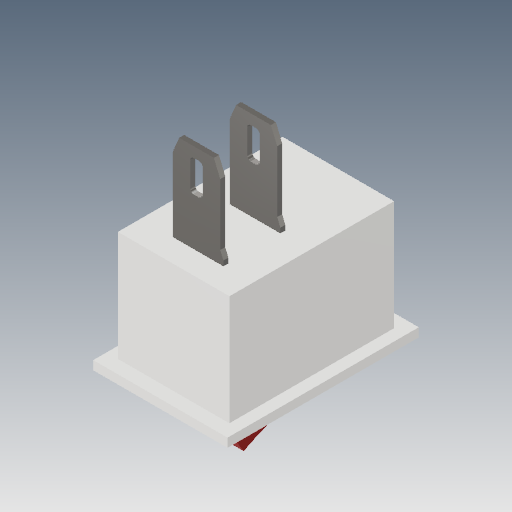
# Autodesk Inventor part: switch_6A
Saved by Autodesk Inventor 2018 (Build 220112000, 112)
## iProperties
Created: 2018-03-28
Part Number: switch_6A
Material: 一般
Document SubType Name: Modeling
Designer: y6tada
Density: 1 g/cm^3
Appearance: 既定
Sending System: SolidWorks 2017
Last Author: y6tada
Last Saved: 2018-06-10
Author: y6tada
Autodesk Inventor part; units mm, degrees
ref_plane "YZ Plane" through (0, 0, 0) normal (1, 0, 0) x (0, 1, 0)
ref_plane "XZ Plane" through (0, 0, 0) normal (0, 1, 0) x (-1, 0, 0)
sketch "スケッチ1" plane through (0, 0, 0) normal (0, 1, 0) x (-1, 0, 0)
  line L0 (4.4, -6.5) -> (-4.4, -6.5)
  line L1 (-4.4, -6.5) -> (-4.4, 6.5)
  line L2 (-4.4, 6.5) -> (4.4, 6.5)
  line L3 (4.4, 6.5) -> (4.4, -6.5)
  line L4 (-4.4, 0) -> (0, 0) construction
  line L5 (0, 0) -> (0, -6.5) construction
  dimension "d0" = 13
  dimension "d1" = 8.8
  constraints: 12 end point, 2 horizontal, 2 midpoint, 2 parallel, 1 perpendicular, 1 vertical
  measures "d0" distance between parallel lines of L2 L0
  measures "d1" distance between parallel lines of L3 L1
extrude "押し出し1" add sketch "スケッチ1" along normal blind 8.7
sketch "スケッチ2" plane through (0, 0, 0) normal (0, -1, 0) x (1, 0, 0)
  line L0 (5.3, 7.55) -> (-5.3, 7.55)
  line L1 (-5.3, 7.55) -> (-5.3, -7.55)
  line L2 (-5.3, -7.55) -> (5.3, -7.55)
  line L3 (5.3, -7.55) -> (5.3, 7.55)
  line L4 (5.3, 0) -> (0, 0) construction
  line L5 (0, 0) -> (0, -7.55) construction
  dimension "d4" = 15.1
  dimension "d5" = 10.6
  constraints: 12 end point, 2 horizontal, 2 midpoint, 2 parallel, 1 perpendicular, 1 vertical
  measures "d4" distance of L0.end L1.end
  measures "d5" distance of L1.end L2.end
extrude "押し出し2" add sketch "スケッチ2" along normal blind 1.5
sketch "スケッチ3" plane through (0, 0, 0) normal (0, 0, 1) x (1, 0, 0)
  line L0 (5.3, -1.5) -> (-5.3, -1.5) construction
  line L1 (-5.3, -1.5) -> (-5.3, -0.7)
  line L2 (-5.3, 0) -> (-5.3, -1.5) construction
  line L3 (-5.3, -0.7) -> (-3.6, -1.5)
  line L4 (-3.6, -1.5) -> (-5.3, -1.5)
  point P0 (0, 0)
  dimension "d8" = 1.7
  dimension "d9" = 0.8
  constraints: 6 end point, 1 perpendicular, 1 point on line
  measures "d8" distance from line of L1 L3.end
  measures "d9" distance of L0.end L1.end
sketch "スケッチ4" plane through (0, -1.5, 0) normal (0, -1, 0) x (1, 0, 0)
  line L0 (5.3, 7.55) -> (-5.3, 7.55) construction
  line L1 (-5.3, 7.55) -> (-5.3, -7.55) construction
  line L2 (-5.3, -7.55) -> (5.3, -7.55) construction
  line L3 (5.3, -7.55) -> (5.3, 7.55) construction
  line L4 (-3.6, 5.85) -> (3.6, 5.85)
  line L5 (3.6, 5.85) -> (3.6, -5.85)
  line L6 (3.6, -5.85) -> (-3.6, -5.85)
  line L7 (-3.6, -5.85) -> (-3.6, 5.85)
  point P0 (0, 0)
  dimension "d10" = 1.7
  constraints: 8 end point, 3 other
  measures "d10" distance between parallel lines of L0 L4
sweep "スイープ1" cut profiles "スケッチ3" path "スケッチ4"
sketch "スケッチ5" plane through (0, 0, 0) normal (1, 0, 0) x (0, 1, 0)
  line L0 (-1.5, 5.85) -> (-1.5, -5.85) construction
  arc A0 (-1.5, -5) -> (-3.75, 4.0973) centre (-21.0161, -5) ccw
  line L1 (-1.5, 5) -> (-1.5, -5)
  line L2 (-21.0161, -5) -> (-1.5, -5) construction
  arc A1 (-1.5, 5) -> (-3.75, 4.0973) centre (-0.8, 0) ccw
  line L3 (-0.8, 0) -> (0, 0) construction
  dimension "d16" = 2.25
  dimension "d17" = 0.8
  dimension "d18" = 10
  constraints: 6 end point, 4 point on circle, 2 centre point, 2 horizontal, 2 point on line, 1 collinear, 1 symmetric about line
  measures "d16" distance from line of L0 A0.end
  measures "d17" distance of L3.start L3.end
  measures "d18" distance of L1.end L1.start
extrude "押し出し3" add sketch "スケッチ5" along normal mid plane 6.25
sketch "スケッチ6" plane through (0, 0, 0) normal (0, 0, 1) x (1, 0, 0)
  line L0 (4.4, 8.7) -> (-4.4, 8.7) construction
  line L1 (0, 8.7) -> (0, 12.8003) construction
  line L2 (-1.875, 8.7) -> (-1.875, 14.55)
  line L3 (-1.875, 14.55) -> (-1.375, 15.75)
  line L4 (-1.375, 15.75) -> (1.375, 15.75)
  line L5 (1.375, 15.75) -> (1.875, 14.55)
  line L6 (1.875, 14.55) -> (1.875, 9.7)
  line L7 (1.875, 9.7) -> (2.125, 9.1)
  line L8 (2.125, 9.1) -> (2.125, 8.7)
  line L9 (2.125, 8.7) -> (-1.875, 8.7)
  line L10 (1.875, 14.55) -> (-1.875, 14.55) construction
  line L11 (0.2, 14.95) -> (-0.2, 14.95)
  line L12 (-0.5, 14.65) -> (-0.5, 12.75)
  line L13 (-0.2, 12.45) -> (0.2, 12.45)
  line L14 (0.5, 12.75) -> (0.5, 14.65)
  arc A0 (0.5, 14.65) -> (0.2, 14.95) centre (0.2, 14.65) ccw
  arc A1 (-0.2, 14.95) -> (-0.5, 14.65) centre (-0.2, 14.65) ccw
  arc A2 (-0.5, 12.75) -> (-0.2, 12.45) centre (-0.2, 12.75) ccw
  arc A3 (0.2, 12.45) -> (0.5, 12.75) centre (0.2, 12.75) ccw
  point P0 (0, 0)
  dimension "d21" = 3.75
  dimension "d22" = 2.75
  dimension "d23" = 1.2
  dimension "d24" = 7.05
  dimension "d25" = 0.25
  dimension "d26" = 0.4
  dimension "d27" = 0.3
  dimension "d28" = 2.5
  dimension "d29" = 1
  dimension "d30" = 0.8
  constraints: 28 end point, 8 point on circle, 8 tangent, 4 centre point, 4 parallel, 3 equal radius, 3 perpendicular, 2 horizontal, 2 point on line, 2 vertical, 1 collinear, 1 midpoint, 1 symmetric about line, 2 other
  measures "d21" distance between parallel lines of L2 L6
  measures "d22" distance of L3.end L4.end
  measures "d23" distance between parallel lines of L10 L4
  measures "d24" distance between parallel lines of L0 L4
  measures "d25" distance between parallel lines of L6 L8
  measures "d26" distance of L7.end L8.end
  measures "d27" radius of A0
  measures "d28" distance between parallel lines of L13 L11
  measures "d29" distance between parallel lines of L14 L12
  measures "d30" distance between parallel lines of L4 L11
extrude "押し出し4" add sketch "スケッチ6" along normal mid plane 0.4
ref_plane "作業平面1" through (0, 0, 4.5) normal (0, 0, 1) x (1, 0, 0)
sketch "スケッチ7" plane through (0, 0, 4.5) normal (0, 0, 1) x (1, 0, 0)
  arc A0 (0.5, 14.65) -> (0.2, 14.95) centre (0.2, 14.65) ccw projected
  line L0 (0.2, 14.95) -> (-0.2, 14.95) projected
  arc A1 (-0.2, 14.95) -> (-0.5, 14.65) centre (-0.2, 14.65) ccw projected
  line L1 (-0.5, 14.65) -> (-0.5, 12.75) projected
  arc A2 (-0.5, 12.75) -> (-0.2, 12.45) centre (-0.2, 12.75) ccw projected
  line L2 (-0.2, 12.45) -> (0.2, 12.45) projected
  arc A3 (0.2, 12.45) -> (0.5, 12.75) centre (0.2, 12.75) ccw projected
  line L3 (0.5, 12.75) -> (0.5, 14.65) projected
  line L4 (-1.875, 8.7) -> (-1.875, 14.55) projected
  line L5 (-1.875, 14.55) -> (-1.375, 15.75) projected
  line L6 (-1.375, 15.75) -> (1.375, 15.75) projected
  line L7 (1.375, 15.75) -> (1.875, 14.55) projected
  line L8 (1.875, 14.55) -> (1.875, 9.7) projected
  line L9 (1.875, 9.7) -> (2.125, 9.1) projected
  line L10 (2.125, 9.1) -> (2.125, 8.7) projected
  line L11 (-1.875, 8.7) -> (2.125, 8.7) projected
  point P0 (0, 0)
extrude "押し出し5" add sketch "スケッチ7" along normal mid plane 0.4
